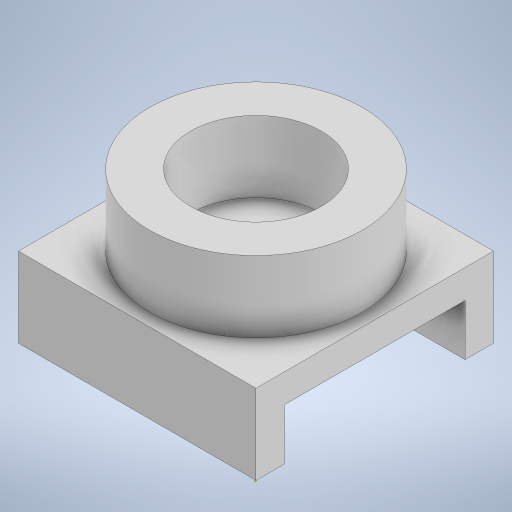
# Autodesk Inventor part: Standard Servo Horn - Linear Holder
Saved by Autodesk Inventor 2023 (Build 270158000, 158)
## iProperties
Created: 2023-09-03
Part Number: Standard Servo Horn - Linear Holder
Material: Generic
Document SubType Name: Modeling
Designer: Nate
Density: 1 g/cm^3
Appearance: Default
Author: Nate
Autodesk Inventor part; units mm, degrees
ref_plane "YZ Plane" through (0, 0, 0) normal (1, 0, 0) x (0, 1, 0)
ref_plane "XZ Plane" through (0, 0, 0) normal (0, 1, 0) x (-1, 0, 0)
ref_plane "XY Plane" through (0, 0, 0) normal (0, 0, 1) x (1, 0, 0)
sketch "Sketch1" plane through (0, 0, 0) normal (0, 1, 0) x (-1, 0, 0)
  line L0 (0, 0) -> (10, 0)
  line L1 (10, 0) -> (10, -10)
  line L2 (10, -10) -> (0, -10)
  line L3 (0, -10) -> (0, 0)
  circle A0 centre (5, -5) radius 4.475
  circle A1 centre (5, -5) radius 2.75
  circle A2 centre (5, -5) radius 1.37
  dimension "d0" = 10
  dimension "d1" = 10
  dimension "d2" = 8.95
  dimension "d3" = 5
  dimension "d4" = 5
  dimension "d5" = 5.5
  dimension "d6" = 2.74
  constraints: 8 end point, 3 centre point, 2 coincident, 2 parallel, 1 horizontal, 1 perpendicular
  measures "d0" distance of L1.end L2.end
  measures "d1" distance of L0.end L1.end
  measures "d2" diameter of A0
  measures "d3" distance from line of L3 A0.centre
  measures "d4" distance from line of A0.centre L0
  measures "d5" diameter of A1
  measures "d6" diameter of A2
extrude "Extrusion1" add sketch "Sketch1" along normal blind 3.36 contours L0 L1 L2 L3
extrude "Extrusion2" add sketch "Sketch1" along normal blind 6.36 contours A0
extrude "Extrusion3" add sketch "Sketch1" along normal blind 3.36 contours A1
sketch "Sketch2" plane through (0, 0, 0) normal (1, 0, 0) x (0, 0, -1)
  line L0 (1.2, 0) -> (8.8, 0)
  line L1 (8.8, 0) -> (8.8, 2.16)
  line L2 (8.8, 2.16) -> (1.2, 2.16)
  line L3 (1.2, 2.16) -> (1.2, 0)
  line L4 (0, 0) -> (10, 0) projected
  dimension "d13" = 7.6
  dimension "d14" = 2.16
  dimension "d15" = 0
  dimension "d16" = 1.2
  constraints: 8 end point, 2 parallel, 1 horizontal, 1 perpendicular
  measures "d13" distance of L2.end L1.end
  measures "d14" distance of L1.end L0.end
  measures "d15" distance between parallel lines of L4 L0
  measures "d16" distance from line of L3 L4.start
extrude "Extrusion4" cut sketch "Sketch2" against normal through all
body "Solid1"
